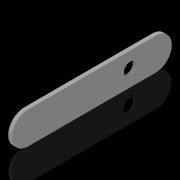
# Autodesk Inventor part: joint
Saved by Autodesk Inventor 2019 (Build 230136000, 136)
## iProperties
Created: 2019-01-06
Part Number: joint
Material: Generic
Document SubType Name: Modeling
Designer: MJ
Density: 1 g/cm^3
Appearance: Default
Author: MJ
Autodesk Inventor part; units mm, degrees
ref_plane "YZ Plane" through (0, 0, 0) normal (1, 0, 0) x (0, 1, 0)
ref_plane "XZ Plane" through (0, 0, 0) normal (0, 1, 0) x (-1, 0, 0)
ref_plane "XY Plane" through (0, 0, 0) normal (0, 0, 1) x (1, 0, 0)
sketch "Sketch1" plane through (0, 0, 0) normal (1, 0, 0) x (0, 1, 0)
  line L0 (0, -25) -> (0, 25) construction
  line L1 (12.5, -25) -> (12.5, 25)
  line L2 (-12.5, 25) -> (-12.5, -25)
  arc A0 (-12.5, -25) -> (12.5, -25) centre (0, -25) ccw
  arc A1 (12.5, 25) -> (-12.5, 25) centre (0, 25) ccw
  line L3 (23.5288, 0) -> (-21.155, 0)
  circle A2 centre (0, 25) radius 5
  circle A3 centre (0, -25) radius 5
  point P0 (0, 0)
  dimension "d1" = 25
  dimension "d15" = 10
  dimension "d16" = 50
  constraints: 10 end point, 4 centre point, 4 point on circle, 4 tangent, 1 coincident, 1 horizontal, 1 midpoint, 1 parallel, 1 point on line, 1 symmetric about line, 1 vertical, 1 other
  measures "d1" diameter of A1
  measures "d15" diameter of A2
  measures "d16" distance of A2.centre A3.centre
extrude "Extrusion1" add sketch "Sketch1" along normal mid plane 3
body "Solid1"
